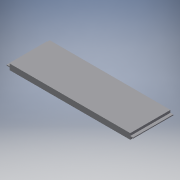
# Autodesk Inventor part: zij
Saved by Autodesk Inventor 2018 (Build 220112000, 112)
## iProperties
Created: 2020-11-10
Part Number: zij
Material: Generic
Document SubType Name: Modeling
Designer: Olivi
Density: 1 g/cm^3
Appearance: Default
Author: Olivi
Autodesk Inventor part; units mm, degrees
ref_plane "YZ Plane" through (0, 0, 0) normal (1, 0, 0) x (0, 1, 0)
ref_plane "XZ Plane" through (0, 0, 0) normal (0, 1, 0) x (-1, 0, 0)
ref_plane "XY Plane" through (0, 0, 0) normal (0, 0, 1) x (1, 0, 0)
sketch "Sketch1" plane through (0, 0, 0) normal (0, 0, 1) x (1, 0, 0)
  line L0 (0, 0) -> (42, 0)
  line L1 (42, 0) -> (42, 14)
  line L2 (42, 14) -> (0, 14)
  line L3 (0, 14) -> (0, 0)
  dimension "d0" = 42
  dimension "d1" = 14
  constraints: 8 end point, 2 parallel, 1 horizontal, 1 perpendicular
  measures "d0" distance of L2.end L1.end
  measures "d1" distance of L1.end L0.end
extrude "Extrusion1" add sketch "Sketch1" along normal blind 2
sketch "Sketch2" plane through (42, 0, 0) normal (1, 0, 0) x (0, 0, -1)
  line L0 (0, 14) -> (-2, 14) projected
  line L1 (-2, 0) -> (-2, 14) projected
  line L2 (0, 0) -> (-2, 0) projected
  line L3 (-1.15, 0) -> (-0.85, 0)
  line L4 (-0.85, 0) -> (-0.85, 14)
  line L5 (-0.85, 14) -> (-1.15, 14)
  line L6 (-1.15, 14) -> (-1.15, 0)
  dimension "d4" = 0.85
  dimension "d5" = 0.3
  constraints: 8 end point, 2 parallel, 2 point on line, 1 horizontal, 1 perpendicular
  measures "d4" distance between parallel lines of L1 L6
  measures "d5" distance between parallel lines of L6 L4
extrude "Extrusion2" add sketch "Sketch2" along normal blind 1 contours L4 L2 L6 L0
sketch "Sketch3" plane through (0, 0, 0) normal (-1, 0, 0) x (0, 0, 1)
  line L0 (0.85, 14) -> (1.15, 14) projected
  line L1 (1.15, 14) -> (1.15, 0) projected
  line L2 (0.85, 14) -> (1.15, 14)
  line L3 (1.15, 14) -> (1.15, 0)
  line L4 (1.15, 0) -> (0.85, 0)
  line L5 (0.85, 0) -> (0.85, 14)
  constraints: 8 end point, 2 parallel, 1 horizontal, 1 perpendicular
extrude "Extrusion3" add sketch "Sketch3" along normal blind 1
body "Solid1"
